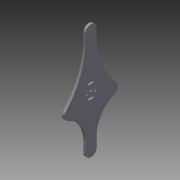
# Autodesk Inventor part: DryRoastedRib
Saved by Autodesk Inventor 2015 (Build 190159000, 159)
## iProperties
Created: 2014-11-09
Part Number: DryRoastedRib
Material: Generic
Document SubType Name: Modeling
Designer: Ryan
Density: 1 g/cm^3
Appearance: Default
Author: Ryan
Autodesk Inventor part; units mm, degrees
ref_plane "YZ Plane" through (0, 0, 0) normal (1, 0, 0) x (0, 1, 0)
ref_plane "XZ Plane" through (0, 0, 0) normal (0, 1, 0) x (-1, 0, 0)
ref_plane "XY Plane" through (0, 0, 0) normal (0, 0, 1) x (1, 0, 0)
sketch "Sketch1" plane through (0, 0, 0) normal (1, 0, 0) x (0, 1, 0)
  line L0 (3.2283, 0) -> (0, 0) construction
  line L1 (0, 0) -> (0, 3.094) construction
  circle A0 centre (0, 0) radius 1.425
  circle A1 centre (70, 0) radius 7.5
  circle A2 centre (-12.5625, 28.6457) radius 7.5
  circle A3 centre (-12.5625, -28.6457) radius 7.5
  circle A4 centre (-70, 0) radius 7.5
  line L2 (70, 0) -> (-12.5625, 28.6457) construction
  line L3 (-12.5625, 28.6457) -> (-12.5625, -28.6457) construction
  line L4 (-12.5625, -28.6457) -> (70, 0) construction
  line L5 (-70, 7.5) -> (-20.0625, 7.5)
  line L6 (-20.0625, 7.5) -> (-20.0625, 28.6457)
  line L7 (-70, -7.5) -> (-20.0625, -7.5)
  line L8 (-20.0625, -7.5) -> (-20.0625, -28.6457)
  line L9 (-5.0625, 28.6457) -> (-5.0625, 7.5)
  line L10 (-5.0625, 7.5) -> (70, 7.5)
  line L11 (70, -7.5) -> (-5.0625, -7.5)
  line L12 (-5.0625, -7.5) -> (-5.0625, -28.6457)
  arc A5 (-7.5202, 34.1977) -> (61.5871, 7.5) centre (61.5871, 110.2914) ccw
  arc A6 (61.5871, -7.5) -> (-7.5202, -34.1977) centre (61.5871, -110.2914) ccw
  arc A7 (-55.7428, 7.5) -> (-19.4724, 31.5616) centre (-55.7428, 46.8677) ccw
  arc A8 (-19.4724, -31.5616) -> (-55.7428, -7.5) centre (-55.7428, -46.8677) ccw
  line L13 (9.9122, 3.55) -> (7.8122, 3.55)
  line L14 (7.8122, 3.55) -> (7.8122, -3.55)
  line L15 (7.8122, -3.55) -> (9.9122, -3.55)
  line L16 (9.9122, -3.55) -> (9.9122, 3.55)
  line L17 (3.5, 6.5) -> (-3.5, 6.5)
  line L18 (-3.5, 6.5) -> (-3.5, 4.5)
  line L19 (-3.5, 4.5) -> (3.5, 4.5)
  line L20 (3.5, 4.5) -> (3.5, 6.5)
  line L21 (-7.8122, 3.55) -> (-9.9122, 3.55)
  line L22 (-9.9122, 3.55) -> (-9.9122, -3.55)
  line L23 (-9.9122, -3.55) -> (-7.8122, -3.55)
  line L24 (-7.8122, -3.55) -> (-7.8122, 3.55)
  line L25 (-3.5, -6.5) -> (3.5, -6.5)
  line L26 (3.5, -6.5) -> (3.5, -4.5)
  line L27 (3.5, -4.5) -> (-3.5, -4.5)
  line L28 (-3.5, -4.5) -> (-3.5, -6.5)
  line L29 (0, 0) -> (-12.5625, -28.6457) construction
  line L30 (0, 0) -> (-12.5625, 21.7589) construction
  line L31 (0, 0) -> (25.125, 0) construction
  line L32 (25.125, 0) -> (-12.5625, 21.7589) construction
  dimension "d2" = 2.85
  dimension "d3" = 15
  dimension "d6" = 15
  dimension "d7" = 140
  dimension "d8" = 2
  dimension "d9" = 2.1
  dimension "d10" = 7
  dimension "d11" = 7.1
  dimension "d12" = 4.5
  dimension "d13" = 7.8122
  dimension "d22" = 25.125
  dimension "d38" = 25.125
  dimension "d39" = 60
  constraints: 66 end point, 20 point on circle, 11 tangent, 9 centre point, 9 horizontal, 8 parallel, 6 point on line, 4 perpendicular, 4 vertical, 1 coincident, 18 other
  measures "d2" diameter of A0
  measures "d3" diameter of A2
  measures "d6" diameter of A1
  measures "d7" distance of A4.centre L2.start
  measures "d8" distance of L19.end L17.start
  measures "d9" distance of L14.end L15.end
  measures "d10" distance of L25.start L25.end
  measures "d11" distance of L15.end L13.start
  measures "d12" distance from line of L19 L0.end
  measures "d13" distance between parallel lines of L24 L1
  measures "d22" distance of L29.start L30.end
  measures "d38" distance of L29.start L31.end
  measures "d39" angle of L3 L32
extrude "Extrusion1" add sketch "Sketch1" along normal blind 3
sketch "Sketch2" plane through (3, 0, 0) normal (1, 0, 0) x (0, 0, -1)
  circle A0 centre (0, 25.125) radius 0.5
  circle A1 centre (-21.7589, -12.5625) radius 0.5
  circle A2 centre (21.7589, -12.5625) radius 0.5
  line L0 (0, 3.9474) -> (0, 0) construction
  line L1 (0, 0) -> (-3.1546, 0) construction
  line L2 (0, 0) -> (-21.7589, -12.5625) construction
  line L3 (0, 0) -> (21.7589, -12.5625) construction
  line L4 (0, 25.125) -> (-21.7589, -12.5625) construction
  line L5 (-21.7589, -12.5625) -> (21.7589, -12.5625) construction
  dimension "d24" = 25.125
  dimension "d26" = 1
  dimension "d27" = 1
  dimension "d28" = 1
  dimension "d29" = 25.125
  dimension "d37" = 60
  constraints: 12 end point, 3 centre point, 2 horizontal, 1 horizontal alignment, 1 symmetric about line, 1 vertical alignment
  measures "d24" distance of L0.end L4.start
  measures "d26" diameter of A0
  measures "d27" diameter of A1
  measures "d28" diameter of A2
  measures "d29" distance of L0.end L2.end
  measures "d37" angle of L5 L4
hole "Hole1" at (3, 25.125, 0) at (3, -12.5625, 21.7589) at (3, -12.5625, -21.7589) direction (-1, 0, 0) diameter 1 end through all
body "Solid1"
